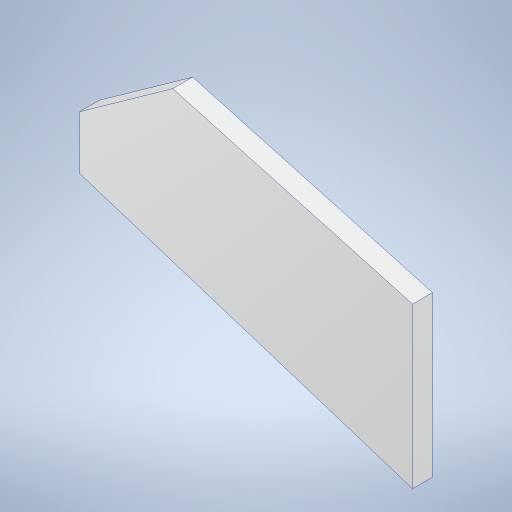
# Autodesk Inventor part: antana_side
Saved by Autodesk Inventor 2024.1 (Build 281209000, 209)
## iProperties
Created: 2024-02-25
Part Number: antana_side
Material: アルミニウム 6061
Document SubType Name: Sheet Metal
Designer: hibik
Density: 2.7 g/cm^3
Sheet Metal Rule: Default_mm
Appearance: アルミニウム - フラット
Author: hibik
Autodesk Inventor part; units mm, degrees
ref_plane "YZ Plane" through (0, 0, 0) normal (1, 0, 0) x (0, 1, 0)
ref_plane "XZ Plane" through (0, 0, 0) normal (0, 1, 0) x (-1, 0, 0)
ref_plane "XY Plane" through (0, 0, 0) normal (0, 0, 1) x (1, 0, 0)
sketch "スケッチ1" plane through (0, 0, 0) normal (0, 0, 1) x (1, 0, 0)
  line L0 (-25, 8) -> (-25, 12)
  line L1 (-25, 12) -> (0, 12)
  line L2 (0, 12) -> (0, 0)
  line L3 (0, 0) -> (-25, 8)
  line L4 (0, 12) -> (-18, 17)
  line L5 (-18, 17) -> (-25, 12)
  dimension "d0" = 12
  dimension "d2" = 4
  dimension "d4" = 25
  dimension "d7" = 5
  dimension "d8" = 18
  measures "d0" distance of L1.end L2.end
  measures "d2" distance of L0.start L0.end
  measures "d4" distance between parallel lines of L2 L0
  measures "d7" distance from line of L1 L4.end
  measures "d8" distance from line of L2 L4.end
extrude "プレート1" add sketch "スケッチ1" along normal blind 1.5
equation "\"d3\" = Thickness"
equation "\"BendRadius\" = Thickness"
equation "\"BendReliefWidth\" = Thickness"
equation "\"BendReliefDepth\" = 0.5 * Thickness"
equation "\"CornerReliefSize\" = 4 * Thickness"
equation "\"MinimumRemnant\" = 2 * Thickness"
equation "\"TransitionRadius\" = BendRadius"
equation "\"JacobiRadiusSize\" = BendRadius"
equation "\"GapSize\" = Thickness"
equation "\"Thickness\" = 1.5"
